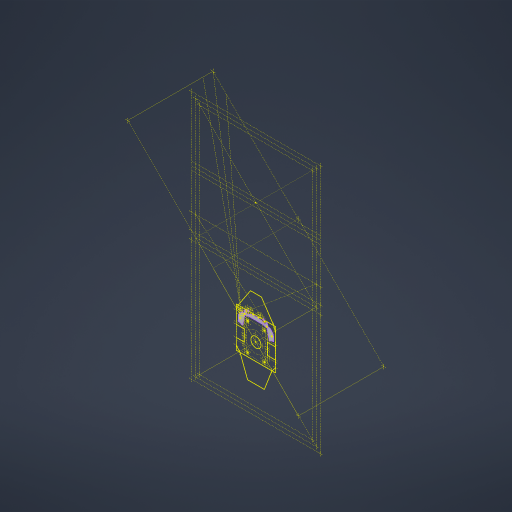
# Autodesk Inventor part: sensorcircuit
Saved by Autodesk Inventor 2023.5 (Build 275446000, 446)
## iProperties
Created: 2025-01-19
Part Number: sensorcircuit
Material: 一般
Document SubType Name: Modeling
Designer: IshiiLabHonda
Density: 1 g/cm^3
Appearance: 既定
Author: IshiiLabHonda
Autodesk Inventor part; units mm, degrees
ref_plane "YZ Plane" through (0, 0, 0) normal (1, 0, 0) x (0, 1, 0)
ref_plane "XZ Plane" through (0, 0, 0) normal (0, 1, 0) x (-1, 0, 0)
ref_plane "XY Plane" through (0, 0, 0) normal (0, 0, 1) x (1, 0, 0)
derived "chassis.ipt"
sketch "スケッチ1" plane through (0, 0, 0) normal (0, 0, 1) x (1, 0, 0)
  line L0 (-90, 90) -> (90, 90) construction
  line L1 (90, 90) -> (90, -90) construction
  line L2 (90, -90) -> (-90, -90) construction
  line L3 (-90, -90) -> (-90, 90) construction
  line L4 (-90, 90) -> (-90, 270) construction
  line L5 (-90, 270) -> (90, 270) construction
  line L6 (90, 270) -> (90, 90) construction
  line L7 (-90, 90) -> (90, -90) construction
  line L8 (90, 90) -> (-90, -90) construction
  line L9 (0, 0) -> (0, 10) construction
  line L10 (0, 0) -> (10, 0) construction
  line L11 (-90, 270) -> (90, 90) construction
  line L12 (-90, 90) -> (90, 270) construction
  line L13 (-96, 276) -> (96, 276) construction
  line L14 (96, 276) -> (96, -96) construction
  line L15 (96, -96) -> (-96, -96) construction
  line L16 (-96, -96) -> (-96, 276) construction
  line L17 (-84, 264) -> (84, 264) construction
  line L18 (84, 264) -> (84, -84) construction
  line L19 (84, -84) -> (-84, -84) construction
  line L20 (-84, -84) -> (-84, 264) construction
  line L21 (-96, 96) -> (96, 96) construction
  line L22 (-96, 84) -> (96, 84) construction
  line L23 (-63.6396, 63.6396) -> (63.6396, 190.9188) construction
  line L24 (63.6396, 190.9188) -> (190.9188, 63.6396) construction
  line L25 (190.9188, 63.6396) -> (63.6396, -63.6396) construction
  line L26 (63.6396, -63.6396) -> (-63.6396, 63.6396) construction
  line L27 (-190.9188, 190.9188) -> (-63.6396, 318.1981) construction
  line L28 (-63.6396, 318.1981) -> (63.6396, 190.9188) construction
  line L29 (-63.6396, 63.6396) -> (-190.9188, 190.9188) construction
  line L30 (-96, 120) -> (96, 120) construction
  line L31 (-96, 186) -> (96, 186) construction
  line L32 (-96, 174) -> (96, 174) construction
  line L33 (-96, 180) -> (96, 180) construction
  point P0 (-63.6396, 318.1981)
  point P1 (-90, 120)
  point P2 (90, 120)
  point P3 (0, 180)
sketch "スケッチ2" plane through (0, 0, 0) normal (0, 0, 1) x (1, 0, 0)
  line L0 (63.6396, 190.9188) -> (190.9188, 63.6396) construction
  line L1 (-63.6396, 318.1981) -> (63.6396, 190.9188) construction
  line L2 (-84, 264) -> (84, 264) construction
  line L3 (-90, 270) -> (90, 270) construction
  line L4 (90, 270) -> (90, 90) construction
  line L5 (-96, 276) -> (96, 276) construction
  line L6 (-90, 90) -> (90, 270) construction
  line L7 (-90, 270) -> (90, 90) construction
  line L8 (-63.6396, 63.6396) -> (63.6396, 190.9188) construction
  line L9 (-96, 120) -> (96, 120) construction
  line L10 (-90, 90) -> (90, 90) construction
  line L11 (-96, 96) -> (96, 96) construction
  line L12 (-96, 84) -> (96, 84) construction
  line L13 (90, -90) -> (-90, -90) construction
  line L14 (0, 0) -> (0, 10) construction
  line L15 (0, 0) -> (10, 0) construction
  line L16 (190.9188, 63.6396) -> (63.6396, -63.6396) construction
  line L17 (63.6396, -63.6396) -> (-63.6396, 63.6396) construction
  line L18 (84, -84) -> (-84, -84) construction
  line L19 (96, -96) -> (-96, -96) construction
  line L20 (-90, 90) -> (-90, 270) construction
  line L21 (-63.6396, 63.6396) -> (-190.9188, 190.9188) construction
  line L22 (-190.9188, 190.9188) -> (-63.6396, 318.1981) construction
  line L23 (96, 276) -> (96, -96) construction
  line L24 (-96, -96) -> (-96, 276) construction
  line L25 (84, 264) -> (84, -84) construction
  line L26 (-84, -84) -> (-84, 264) construction
  line L27 (90, 90) -> (90, -90) construction
  line L28 (-90, 90) -> (90, -90) construction
  line L29 (90, 90) -> (-90, -90) construction
  line L30 (-90, -90) -> (-90, 90) construction
  circle A0 centre (0, 0) radius 15 construction
  circle A1 centre (0, 0) radius 7.5 construction
  line L31 (20, 11.5) -> (28.75, 11.5) construction
  line L32 (28.75, 11.5) -> (28.75, -11.5) construction
  line L33 (28.75, -11.5) -> (20, -11.5) construction
  line L34 (20, -11.5) -> (20, 11.5) construction
  line L35 (20, 11.5) -> (18, 11.5) construction
  line L36 (18, 11.5) -> (18, -11.5) construction
  line L37 (18, -11.5) -> (20, -11.5) construction
  line L38 (18, 1.5) -> (17, 1.5) construction
  line L39 (17, -1.5) -> (18, -1.5) construction
  line L40 (-17, 24) -> (17, 24) construction
  line L41 (17, 24) -> (17, -22) construction
  line L42 (17, -22) -> (-17, -22) construction
  line L43 (-17, -22) -> (-17, 24) construction
  line L44 (-20, 11.5) -> (-18, 11.5) construction
  line L45 (-17, -1.5) -> (-18, -1.5) construction
  line L46 (-20, -11.5) -> (-20, 11.5) construction
  line L47 (-18, 11.5) -> (-18, -11.5) construction
  line L48 (-28.75, -11.5) -> (-20, -11.5) construction
  line L49 (-20, 11.5) -> (-28.75, 11.5) construction
  line L50 (-28.75, 11.5) -> (-28.75, -11.5) construction
  line L51 (-18, -11.5) -> (-20, -11.5) construction
  line L52 (-18, 1.5) -> (-17, 1.5) construction
  line L53 (-14.5, 24) -> (-14.5, -22) construction
  line L54 (14.5, 24) -> (14.5, -22) construction
  line L55 (-10.5, 24) -> (-10.5, 19) construction
  line L56 (-10.5, 19) -> (-14.5, 19) construction
  line L57 (-14.5, 24) -> (-10.5, 19) construction
  line L58 (-10.5, 24) -> (-14.5, 19) construction
  circle A2 centre (-12.5, 21.5) radius 1 construction
  line L59 (10.5, 24) -> (10.5, 19) construction
  line L60 (10.5, 19) -> (14.5, 19) construction
  line L61 (10.5, 24) -> (14.5, 19) construction
  line L62 (10.5, 19) -> (14.5, 24) construction
  circle A3 centre (12.5, 21.5) radius 1 construction
  line L63 (-14.5, -17) -> (-10.5, -17) construction
  line L64 (-10.5, -17) -> (-10.5, -22) construction
  line L65 (10.5, -22) -> (10.5, -17) construction
  line L66 (10.5, -17) -> (14.5, -17) construction
  line L67 (-14.5, -17) -> (-10.5, -22) construction
  line L68 (-10.5, -17) -> (-14.5, -22) construction
  circle A4 centre (-12.5, -19.5) radius 1 construction
  line L69 (10.5, -17) -> (14.5, -22) construction
  line L70 (14.5, -17) -> (10.5, -22) construction
  circle A5 centre (12.5, -19.5) radius 1 construction
  point P0 (90, 120)
  point P1 (-90, 120)
  point P2 (-63.6396, 318.1981)
  point P3 (-12.5, -19.5)
sketch "スケッチ3" plane through (0, 0, 0) normal (0, 0, 1) x (1, 0, 0)
  line L0 (63.6396, 190.9188) -> (190.9188, 63.6396) construction
  line L1 (-63.6396, 318.1981) -> (63.6396, 190.9188) construction
  line L2 (-84, 264) -> (84, 264) construction
  line L3 (-90, 270) -> (90, 270) construction
  line L4 (90, 270) -> (90, 90) construction
  line L5 (-96, 276) -> (96, 276) construction
  line L6 (-90, 90) -> (90, 270) construction
  line L7 (-90, 270) -> (90, 90) construction
  line L8 (-63.6396, 63.6396) -> (63.6396, 190.9188) construction
  line L9 (-96, 120) -> (96, 120) construction
  line L10 (-90, 90) -> (90, 90) construction
  line L11 (-96, 96) -> (96, 96) construction
  line L12 (-96, 84) -> (96, 84) construction
  line L13 (90, -90) -> (-90, -90) construction
  line L14 (0, 0) -> (0, 10) construction
  line L15 (0, 0) -> (10, 0) construction
  line L16 (190.9188, 63.6396) -> (63.6396, -63.6396) construction
  line L17 (63.6396, -63.6396) -> (-63.6396, 63.6396) construction
  line L18 (84, -84) -> (-84, -84) construction
  line L19 (96, -96) -> (-96, -96) construction
  line L20 (-90, 90) -> (-90, 270) construction
  line L21 (-63.6396, 63.6396) -> (-190.9188, 190.9188) construction
  line L22 (-190.9188, 190.9188) -> (-63.6396, 318.1981) construction
  line L23 (96, 276) -> (96, -96) construction
  line L24 (-96, -96) -> (-96, 276) construction
  line L25 (84, 264) -> (84, -84) construction
  line L26 (-84, -84) -> (-84, 264) construction
  line L27 (90, 90) -> (90, -90) construction
  line L28 (-90, 90) -> (90, -90) construction
  line L29 (90, 90) -> (-90, -90) construction
  line L30 (-90, -90) -> (-90, 90) construction
  line L31 (-18, 1.5) -> (-17, 1.5) construction
  line L32 (-17, -1.5) -> (-18, -1.5) construction
  line L33 (-20, 11.5) -> (-18, 11.5) construction
  line L34 (-28.75, 11.5) -> (-28.75, -11.5) construction
  line L35 (63.6396, -63.6396) -> (-63.6396, 63.6396) construction
  line L36 (84, -84) -> (-84, -84) construction
  line L37 (-90, -90) -> (-90, 90) construction
  line L38 (96, -96) -> (-96, -96) construction
  line L39 (-90, 90) -> (90, 90) construction
  line L40 (90, -90) -> (-90, -90) construction
  line L41 (90, 90) -> (-90, -90) construction
  line L42 (-90, 90) -> (90, -90) construction
  line L43 (90, 90) -> (90, -90) construction
  line L44 (-28.75, -11.5) -> (-20, -11.5) construction
  line L45 (-20, 11.5) -> (-28.75, 11.5) construction
  line L46 (-18, 11.5) -> (-18, -11.5) construction
  line L47 (-18, -11.5) -> (-20, -11.5) construction
  line L48 (0, 0) -> (0, 10) construction
  line L49 (0, 0) -> (10, 0) construction
  circle A0 centre (0, 0) radius 15 construction
  circle A1 centre (0, 0) radius 7.5
  line L50 (-14.5, 24) -> (-14.5, -22) construction
  line L51 (-17, 24) -> (17, 24) construction
  line L52 (-17, -22) -> (-17, 24) construction
  line L53 (17, -22) -> (-17, -22) construction
  line L54 (-14.5, -17) -> (-10.5, -17) construction
  circle A2 centre (-12.5, -19.5) radius 1
  line L55 (-10.5, -17) -> (-14.5, -22) construction
  line L56 (-14.5, -17) -> (-10.5, -22) construction
  line L57 (-63.6396, 318.1981) -> (63.6396, 190.9188) construction
  line L58 (-84, 264) -> (84, 264) construction
  line L59 (-90, 270) -> (90, 270) construction
  line L60 (90, 270) -> (90, 90) construction
  line L61 (-96, 276) -> (96, 276) construction
  line L62 (-90, 90) -> (90, 270) construction
  line L63 (-90, 270) -> (90, 90) construction
  line L64 (-63.6396, 63.6396) -> (63.6396, 190.9188) construction
  line L65 (-96, 120) -> (96, 120) construction
  line L66 (-96, 96) -> (96, 96) construction
  line L67 (-96, 84) -> (96, 84) construction
  line L68 (84, 264) -> (84, -84) construction
  line L69 (96, 276) -> (96, -96) construction
  line L70 (-96, -96) -> (-96, 276) construction
  line L71 (-84, -84) -> (-84, 264) construction
  line L72 (-63.6396, 63.6396) -> (-190.9188, 190.9188) construction
  line L73 (-90, 90) -> (-90, 270) construction
  line L74 (-190.9188, 190.9188) -> (-63.6396, 318.1981) construction
  line L75 (-20, -11.5) -> (-20, 11.5) construction
  line L76 (10.5, -17) -> (14.5, -17) construction
  line L77 (10.5, -22) -> (10.5, -17) construction
  circle A3 centre (12.5, -19.5) radius 1
  line L78 (10.5, -17) -> (14.5, -22) construction
  line L79 (14.5, -17) -> (10.5, -22) construction
  line L80 (-10.5, -17) -> (-10.5, -22) construction
  line L81 (63.6396, 190.9188) -> (190.9188, 63.6396) construction
  line L82 (190.9188, 63.6396) -> (63.6396, -63.6396) construction
  line L83 (20, 11.5) -> (28.75, 11.5) construction
  line L84 (28.75, 11.5) -> (28.75, -11.5) construction
  line L85 (17, -1.5) -> (18, -1.5) construction
  line L86 (18, -11.5) -> (20, -11.5) construction
  line L87 (28.75, -11.5) -> (20, -11.5) construction
  line L88 (14.5, 24) -> (14.5, -22) construction
  line L89 (17, 24) -> (17, -22) construction
  line L90 (18, 11.5) -> (18, -11.5) construction
  line L91 (20, -11.5) -> (20, 11.5) construction
  line L92 (20, 11.5) -> (18, 11.5) construction
  line L93 (18, 1.5) -> (17, 1.5) construction
  line L94 (-10.5, 24) -> (-10.5, 19) construction
  line L95 (10.5, 19) -> (14.5, 19) construction
  circle A4 centre (12.5, 21.5) radius 1
  line L96 (10.5, 24) -> (14.5, 19) construction
  line L97 (10.5, 19) -> (14.5, 24) construction
  line L98 (10.5, 24) -> (10.5, 19) construction
  line L99 (-10.5, 19) -> (-14.5, 19) construction
  circle A5 centre (-12.5, 21.5) radius 1
  line L100 (-14.5, 24) -> (-10.5, 19) construction
  line L101 (-10.5, 24) -> (-14.5, 19) construction
  line L102 (-29.25, 34.7741) -> (29.25, 34.7741)
  line L103 (29.25, 34.7741) -> (29.25, -25)
  line L104 (29.25, -25) -> (-29.25, -25)
  line L105 (-29.25, -25) -> (-29.25, 34.7741)
  line L106 (-29.25, 8.5) -> (-17, 8.5)
  line L107 (-17, 8.5) -> (-17, -8.5)
  line L108 (-17, -8.5) -> (-29.25, -8.5)
  line L109 (29.25, 8.5) -> (17, 8.5)
  line L110 (17, 8.5) -> (17, -8.5)
  line L111 (17, -8.5) -> (29.25, -8.5)
  line L112 (-19.2916, 33.0498) -> (-18.0519, 24.3881) construction
  line L113 (4.1489, 37.7362) -> (7.3628, 41.5664) construction
  line L114 (2.9316, 37.4522) -> (7.4311, 42.8145) construction
  line L115 (7.9109, 33.2741) -> (2.9316, 37.4522) construction
  line L116 (7.4311, 42.8145) -> (7.9109, 33.2741) construction
  line L117 (7.9791, 34.5222) -> (7.3628, 41.5664) construction
  line L118 (7.9791, 34.5222) -> (4.1489, 37.7362) construction
  line L119 (7.9109, 33.2741) -> (10.209, 31.3457) construction
  line L120 (7.3628, 41.5664) -> (11.1931, 38.3525) construction
  line L121 (4.1489, 37.7362) -> (11.1931, 38.3525) construction
  line L122 (11.1931, 38.3525) -> (7.9791, 34.5222) construction
  line L123 (2.9316, 37.4522) -> (12.4104, 38.6364) construction
  line L124 (7.4311, 42.8145) -> (12.4104, 38.6364) construction
  line L125 (12.4104, 38.6364) -> (7.9109, 33.2741) construction
  line L126 (10.209, 31.3457) -> (14.7085, 36.7081) construction
  line L127 (14.7085, 36.7081) -> (12.4104, 38.6364) construction
  line L128 (-16.0041, 31.7777) -> (-14.4163, 27.8774) construction
  line L129 (-20.1753, 32.1657) -> (-14.4163, 27.8774) construction
  line L130 (-19.4669, 27.2161) -> (-16.0041, 31.7777) construction
  line L131 (-20.1753, 32.1657) -> (-19.4669, 27.2161) construction
  line L132 (-22.2959, 29.3367) -> (-17.2502, 30.0278) construction
  line L133 (-25.1248, 31.4573) -> (-16.0041, 31.7777) construction
  line L134 (-25.1248, 31.4573) -> (-19.4669, 27.2161) construction
  line L135 (-14.4163, 27.8774) -> (-24.4164, 26.5077) construction
  line L136 (-24.4164, 26.5077) -> (-20.1753, 32.1657) construction
  line L137 (-26.221, 32.058) -> (-19.2916, 33.0498) construction
  line L138 (-24.4164, 26.5077) -> (-25.1248, 31.4573) construction
  line L139 (-18.0519, 24.3881) -> (-24.9813, 23.3963) construction
  line L140 (-24.9813, 23.3963) -> (-26.221, 32.058) construction
  line L141 (-63.6396, 318.1981) -> (-22.2959, 29.3367) construction
  line L142 (7.671, 38.0443) -> (-90, 120) construction
  line L143 (-22.2959, 29.3367) -> (-78.7203, 303.1174) construction
  line L144 (-22.2959, 29.3367) -> (-44.186, 298.7444) construction
  line L145 (-7.671, 38.0443) -> (90, 120) construction
  line L146 (-7.3628, 41.5664) -> (-4.1489, 37.7362) construction
  line L147 (-7.4311, 42.8145) -> (-2.9316, 37.4522) construction
  line L148 (-12.4104, 38.6364) -> (-7.4311, 42.8145) construction
  line L149 (-2.9316, 37.4522) -> (-12.4104, 38.6364) construction
  line L150 (-11.1931, 38.3525) -> (-4.1489, 37.7362) construction
  line L151 (-11.1931, 38.3525) -> (-7.3628, 41.5664) construction
  line L152 (-12.4104, 38.6364) -> (-14.7085, 36.7081) construction
  line L153 (-4.1489, 37.7362) -> (-7.9791, 34.5222) construction
  line L154 (-7.3628, 41.5664) -> (-7.9791, 34.5222) construction
  line L155 (-7.4311, 42.8145) -> (-7.9109, 33.2741) construction
  line L156 (-2.9316, 37.4522) -> (-7.9109, 33.2741) construction
  line L157 (-7.9109, 33.2741) -> (-12.4104, 38.6364) construction
  line L158 (-14.7085, 36.7081) -> (-10.209, 31.3457) construction
  line L159 (-10.209, 31.3457) -> (-7.9109, 33.2741) construction
  line L160 (-7.9791, 34.5222) -> (-11.1931, 38.3525) construction
  line L161 (-26.6098, 34.7741) -> (-29.25, 26.6905)
  line L162 (26.6098, 34.7741) -> (29.25, 26.6905)
  line L163 (-29.25, -18.5) -> (-23.7959, -25)
  line L164 (23.7959, -25) -> (29.25, -18.5)
  circle A6 centre (-3.9665, 33.6295) radius 0.625
  circle A7 centre (-3.9665, 33.6295) radius 0.8 construction
  circle A8 centre (-3.9665, 33.6295) radius 1.5 construction
  circle A9 centre (-13.3559, 33.2741) radius 1.5 construction
  circle A10 centre (-13.3559, 33.2741) radius 0.8 construction
  circle A11 centre (-13.3559, 33.2741) radius 0.625
  circle A12 centre (-11.4763, 34.8513) radius 1.1616
  circle A13 centre (11.4763, 34.8513) radius 1.1833
  line L165 (-19.4669, 27.2161) -> (-24.4164, 26.5077) construction
  line L166 (-25.3001, 25.6236) -> (-18.3707, 26.6154) construction
  line L167 (-24.7706, 28.9825) -> (-19.8211, 29.6909) construction
  line L168 (-21.5166, 23.8922) -> (-21.9416, 26.8619) construction
  circle A14 centre (-23.7959, 19.3461) radius 0.625 construction
  circle A15 centre (-23.7959, 19.3461) radius 0.8
  circle A16 centre (-23.7959, 19.3461) radius 1.5 construction
  circle A17 centre (-16.474, 28.323) radius 0.625 construction
  circle A18 centre (-16.474, 28.323) radius 0.8
  circle A19 centre (-16.474, 28.323) radius 1.5 construction
  line L169 (-25.1248, 31.4573) -> (-20.1753, 32.1657) construction
  line L170 (-23.7959, -25) -> (-12.5, -54.725)
  line L171 (-12.5, -54.725) -> (12.5, -54.725)
  line L172 (12.5, -54.725) -> (23.7959, -25)
  line L173 (-26.6098, 34.7741) -> (-8.142, 62.5133)
  line L174 (-8.142, 62.5133) -> (8.1348, 62.5133)
  line L175 (8.1348, 62.5133) -> (26.6098, 34.7741)
  circle A20 centre (23.7959, 19.3461) radius 0.625 construction
  circle A21 centre (23.7959, 19.3461) radius 0.8
  circle A22 centre (23.7959, 19.3461) radius 1.5 construction
  circle A23 centre (16.474, 28.323) radius 0.625 construction
  circle A24 centre (16.474, 28.323) radius 0.8
  circle A25 centre (16.474, 28.323) radius 1.5 construction
  circle A26 centre (13.3559, 33.2741) radius 1.5 construction
  circle A27 centre (13.3559, 33.2741) radius 0.625 construction
  circle A28 centre (13.3559, 33.2741) radius 0.8
  circle A29 centre (3.9665, 33.6295) radius 1.5 construction
  circle A30 centre (3.9665, 33.6295) radius 0.8
  circle A31 centre (3.9665, 33.6295) radius 0.625 construction
  point P0 (-22.2959, 29.3367)
  point P1 (-22.2959, 29.3367)
sketch "スケッチ4" plane through (0, 0, 0) normal (0, 0, 1) x (1, 0, 0)
  line L0 (-20, 11.5) -> (-28.75, 11.5) construction
  line L1 (-28.75, 11.5) -> (-28.75, -11.5) construction
  line L2 (-28.75, -11.5) -> (-20, -11.5) construction
  line L3 (20, 11.5) -> (28.75, 11.5) construction
  line L4 (18, 1.5) -> (17, 1.5) construction
  line L5 (17, -1.5) -> (18, -1.5) construction
  line L6 (18, -11.5) -> (20, -11.5) construction
  line L7 (18, 11.5) -> (18, -11.5) construction
  line L8 (14.5, 24) -> (14.5, -22) construction
  line L9 (17, 24) -> (17, -22) construction
  line L10 (20, 11.5) -> (18, 11.5) construction
  line L11 (20, -11.5) -> (20, 11.5) construction
  line L12 (28.75, -11.5) -> (20, -11.5) construction
  line L13 (28.75, 11.5) -> (28.75, -11.5) construction
  line L14 (0, 0) -> (0, 10) construction
  line L15 (0, 0) -> (10, 0) construction
  circle A0 centre (0, 0) radius 15 construction
  circle A1 centre (0, 0) radius 7.5 construction
  line L16 (-17, 24) -> (17, 24) construction
  line L17 (17, -22) -> (-17, -22) construction
  line L18 (-14.5, 24) -> (-14.5, -22) construction
  line L19 (-17, -22) -> (-17, 24) construction
  line L20 (-18, 11.5) -> (-18, -11.5) construction
  line L21 (-20, -11.5) -> (-20, 11.5) construction
  line L22 (-18, 1.5) -> (-17, 1.5) construction
  line L23 (-18, -11.5) -> (-20, -11.5) construction
  line L24 (-17, -1.5) -> (-18, -1.5) construction
  line L25 (-10.5, 19) -> (-14.5, 19) construction
  line L26 (-10.5, 24) -> (-10.5, 19) construction
  line L27 (-10.5, 24) -> (-14.5, 19) construction
  line L28 (-14.5, 24) -> (-10.5, 19) construction
  line L29 (-20, 11.5) -> (-18, 11.5) construction
  circle A2 centre (-12.5, 21.5) radius 1 construction
  line L30 (-14.5, -17) -> (-10.5, -17) construction
  circle A3 centre (-12.5, -19.5) radius 1 construction
  line L31 (-14.5, -17) -> (-10.5, -22) construction
  line L32 (-10.5, -17) -> (-14.5, -22) construction
  line L33 (-10.5, -17) -> (-10.5, -22) construction
  line L34 (10.5, -17) -> (14.5, -17) construction
  circle A4 centre (12.5, -19.5) radius 1 construction
  line L35 (10.5, -22) -> (10.5, -17) construction
  line L36 (10.5, -17) -> (14.5, -22) construction
  line L37 (14.5, -17) -> (10.5, -22) construction
  line L38 (10.5, 19) -> (14.5, 19) construction
  circle A5 centre (12.5, 21.5) radius 1 construction
  line L39 (10.5, 24) -> (14.5, 19) construction
  line L40 (10.5, 19) -> (14.5, 24) construction
  line L41 (10.5, 24) -> (10.5, 19) construction
  line L42 (0, 0) -> (0, 10) construction
  line L43 (0, 0) -> (10, 0) construction
  line L44 (0, 0) -> (0, 10) construction
  line L45 (0, 0) -> (10, 0) construction
  line L46 (10.5, -22) -> (10.5, -17) construction
  line L47 (17, -1.5) -> (18, -1.5) construction
  line L48 (18, 1.5) -> (17, 1.5) construction
  line L49 (20, -11.5) -> (20, 11.5) construction
  line L50 (18, 11.5) -> (18, -11.5) construction
  line L51 (28.75, 11.5) -> (28.75, -11.5) construction
  line L52 (-10.5, -17) -> (-10.5, -22) construction
  line L53 (10.5, 19) -> (14.5, 19) construction
  circle A6 centre (12.5, 21.5) radius 1 projected
  line L54 (-17, -1.5) -> (-18, -1.5) construction
  line L55 (14.5, 24) -> (14.5, -22) construction
  line L56 (10.5, 24) -> (14.5, 19) construction
  line L57 (10.5, 19) -> (14.5, 24) construction
  line L58 (17, 24) -> (17, -22) construction
  line L59 (10.5, 24) -> (10.5, 19) construction
  line L60 (-18, 1.5) -> (-17, 1.5) construction
  line L61 (-17, 8.5) -> (-17, -8.5) projected
  line L62 (-20, 11.5) -> (-18, 11.5) construction
  line L63 (-20, -11.5) -> (-20, 11.5) construction
  line L64 (29.25, 34.7741) -> (29.25, -25) projected
  line L65 (-29.25, -25) -> (-29.25, 34.7741) projected
  line L66 (-28.75, 11.5) -> (-28.75, -11.5) construction
  line L67 (18, -11.5) -> (20, -11.5) construction
  line L68 (10.5, -17) -> (14.5, -17) construction
  line L69 (28.75, -11.5) -> (20, -11.5) construction
  line L70 (10.5, -17) -> (14.5, -22) construction
  line L71 (20, 11.5) -> (18, 11.5) construction
  line L72 (29.25, 8.5) -> (17, 8.5) projected
  line L73 (20, 11.5) -> (28.75, 11.5) construction
  line L74 (17, 8.5) -> (17, -8.5) projected
  line L75 (-20, 11.5) -> (-28.75, 11.5) construction
  line L76 (7.4311, 42.8145) -> (12.4104, 38.6364) construction
  line L77 (7.9109, 33.2741) -> (10.209, 31.3457) construction
  line L78 (10.209, 31.3457) -> (14.7085, 36.7081) construction
  line L79 (7.9791, 34.5222) -> (7.3628, 41.5664) construction
  line L80 (4.1489, 37.7362) -> (7.3628, 41.5664) construction
  line L81 (2.9316, 37.4522) -> (7.4311, 42.8145) construction
  line L82 (7.9791, 34.5222) -> (4.1489, 37.7362) construction
  circle A7 centre (11.4763, 34.8513) radius 1.1833 projected
  line L83 (7.9109, 33.2741) -> (2.9316, 37.4522) construction
  line L84 (7.4311, 42.8145) -> (7.9109, 33.2741) construction
  line L85 (4.1489, 37.7362) -> (11.1931, 38.3525) construction
  line L86 (2.9316, 37.4522) -> (12.4104, 38.6364) construction
  line L87 (7.3628, 41.5664) -> (11.1931, 38.3525) construction
  line L88 (11.1931, 38.3525) -> (7.9791, 34.5222) construction
  line L89 (12.4104, 38.6364) -> (7.9109, 33.2741) construction
  line L90 (14.7085, 36.7081) -> (12.4104, 38.6364) construction
  line L91 (26.6098, 34.7741) -> (29.25, 26.6905) projected
  circle A8 centre (-12.5, 21.5) radius 1 projected
  line L92 (-10.5, 19) -> (-14.5, 19) construction
  line L93 (-10.5, 24) -> (-10.5, 19) construction
  line L94 (-14.5, 24) -> (-10.5, 19) construction
  line L95 (-10.5, 24) -> (-14.5, 19) construction
  line L96 (-22.2959, 29.3367) -> (-17.2502, 30.0278) construction
  line L97 (-14.4163, 27.8774) -> (-24.4164, 26.5077) construction
  line L98 (-24.4164, 26.5077) -> (-25.1248, 31.4573) construction
  line L99 (-20.1753, 32.1657) -> (-14.4163, 27.8774) construction
  line L100 (-20.1753, 32.1657) -> (-19.4669, 27.2161) construction
  line L101 (-24.4164, 26.5077) -> (-20.1753, 32.1657) construction
  line L102 (-25.1248, 31.4573) -> (-19.4669, 27.2161) construction
  line L103 (-18.0519, 24.3881) -> (-24.9813, 23.3963) construction
  line L104 (-25.1248, 31.4573) -> (-16.0041, 31.7777) construction
  line L105 (-16.0041, 31.7777) -> (-14.4163, 27.8774) construction
  line L106 (-19.4669, 27.2161) -> (-16.0041, 31.7777) construction
  line L107 (-19.2916, 33.0498) -> (-18.0519, 24.3881) construction
  line L108 (-26.221, 32.058) -> (-19.2916, 33.0498) construction
  line L109 (-24.9813, 23.3963) -> (-26.221, 32.058) construction
  line L110 (-28.75, -11.5) -> (-20, -11.5) construction
  line L111 (-29.25, 8.5) -> (-17, 8.5) projected
  line L112 (-10.209, 31.3457) -> (-7.9109, 33.2741) construction
  circle A9 centre (-13.3559, 33.2741) radius 0.625 projected
  circle A10 centre (-13.3559, 33.2741) radius 0.8 construction
  circle A11 centre (-13.3559, 33.2741) radius 1.5 construction
  line L113 (-14.7085, 36.7081) -> (-10.209, 31.3457) construction
  line L114 (-2.9316, 37.4522) -> (-7.9109, 33.2741) construction
  line L115 (-4.1489, 37.7362) -> (-7.9791, 34.5222) construction
  line L116 (-2.9316, 37.4522) -> (-12.4104, 38.6364) construction
  line L117 (-11.1931, 38.3525) -> (-4.1489, 37.7362) construction
  line L118 (-7.9791, 34.5222) -> (-11.1931, 38.3525) construction
  line L119 (-12.4104, 38.6364) -> (-14.7085, 36.7081) construction
  line L120 (-7.9109, 33.2741) -> (-12.4104, 38.6364) construction
  circle A12 centre (-11.4763, 34.8513) radius 1.1616 projected
  line L121 (-11.1931, 38.3525) -> (-7.3628, 41.5664) construction
  line L122 (-7.3628, 41.5664) -> (-7.9791, 34.5222) construction
  line L123 (-12.4104, 38.6364) -> (-7.4311, 42.8145) construction
  line L124 (-7.4311, 42.8145) -> (-7.9109, 33.2741) construction
  line L125 (-26.6098, 34.7741) -> (-29.25, 26.6905) projected
  line L126 (0, 0) -> (0, 10) construction
  line L127 (0, 0) -> (10, 0) construction
  circle A13 centre (0, 0) radius 7.5 projected
  line L128 (-14.5, -17) -> (-10.5, -17) construction
  circle A14 centre (0, 0) radius 15 construction
  circle A15 centre (12.5, -19.5) radius 1 projected
  line L129 (14.5, -17) -> (10.5, -22) construction
  circle A16 centre (-12.5, -19.5) radius 1 projected
  line L130 (-14.5, -17) -> (-10.5, -22) construction
  line L131 (17, -22) -> (-17, -22) construction
  line L132 (-29.25, 34.7741) -> (29.25, 34.7741) projected
  line L133 (23.7959, -25) -> (29.25, -18.5) projected
  line L134 (-29.25, -18.5) -> (-23.7959, -25) projected
  line L135 (29.25, -25) -> (-29.25, -25) projected
  line L136 (-17, -8.5) -> (-29.25, -8.5) projected
  line L137 (-18, -11.5) -> (-20, -11.5) construction
  line L138 (-18, 11.5) -> (-18, -11.5) construction
  circle A17 centre (-3.9665, 33.6295) radius 0.625 projected
  circle A18 centre (-3.9665, 33.6295) radius 1.5 construction
  line L139 (-7.3628, 41.5664) -> (-4.1489, 37.7362) construction
  line L140 (-7.4311, 42.8145) -> (-2.9316, 37.4522) construction
  circle A19 centre (-3.9665, 33.6295) radius 0.8 construction
  line L141 (-10.5, -17) -> (-14.5, -22) construction
  line L142 (-14.5, 24) -> (-14.5, -22) construction
  line L143 (-17, -22) -> (-17, 24) construction
  line L144 (-17, 24) -> (17, 24) construction
  line L145 (17, -8.5) -> (29.25, -8.5) projected
  line L146 (-10.9787, 28.0539) -> (-12.6578, 27.2854)
  line L147 (-12.6578, 27.2854) -> (-16.5, 26.9)
  line L148 (-16.5, 26.9) -> (-19.7538, 12.1943)
  line L149 (-19.7538, 12.1943) -> (-26.6159, 14.1073)
  line L150 (-10.9787, 28.0539) -> (0, 28.0539)
  line L151 (-26.6159, 14.1073) -> (-26.0632, 22.8433)
  line L152 (-26.0632, 22.8433) -> (-21.4258, 28.4547)
  line L153 (-21.4258, 28.4547) -> (-18.0818, 29.0596)
  line L154 (-6.915, 32.35) -> (0, 33.078)
  line L155 (10.9787, 28.0539) -> (12.6578, 27.2854)
  line L156 (12.6578, 27.2854) -> (16.5, 26.9)
  line L157 (16.5, 26.9) -> (19.7538, 12.1943)
  line L158 (19.7538, 12.1943) -> (26.6159, 14.1073)
  line L159 (10.9787, 28.0539) -> (0, 28.0539)
  line L160 (26.6159, 14.1073) -> (26.0632, 22.8433)
  line L161 (26.0632, 22.8433) -> (21.4258, 28.4547)
  line L162 (21.4258, 28.4547) -> (18.0818, 29.0596)
  line L163 (6.915, 32.35) -> (0, 33.078)
  line L164 (-16.5, 34.4151) -> (-13.4256, 29.902)
  line L165 (-13.4256, 29.902) -> (-6.915, 32.35)
  line L166 (-18.0818, 29.0596) -> (-16.5, 34.4151)
  line L167 (16.5, 34.4151) -> (13.4256, 29.902)
  line L168 (18.0818, 29.0596) -> (16.5, 34.4151)
  line L169 (6.915, 32.35) -> (13.4256, 29.902)
  point P0 (-12.5, -19.5)
  point P1 (7.671, 38.0443)
  point P2 (-22.2959, 29.3367)
  point P3 (-7.671, 38.0443)
  constraints: 48 end point, 11 horizontal alignment, 25 other
extrude "押し出し1" add sketch "スケッチ4" against normal blind 0.6 contours L146 L147 L148 L149 L151 L152 L153 L166 L164 L165 L154 L163 L169 L167 L168 L162 L161 L160 L158 L157 L156 L155 L159 L150
